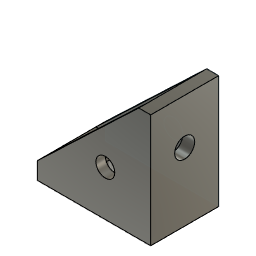
2020_CornerCube-18mm (Autodesk Fusion 360 design; units mm, degrees)
Autodesk Fusion 360 part; units mm, degrees
sketch "スケッチ1" plane through (0, 0, 0) normal (1, 0, 0) x (0, 1, 0)
  line L0 (0, 0) -> (0, 30)
  line L1 (0, 0) -> (30, 0)
  line L2 (30, 0) -> (0, 30)
  constraint coincident L0.start L1.start
  constraint vertical L0
  constraint perpendicular L0 L1
sketch "スケッチ2" plane through (0, 0, 0) normal (1, 0, 0) x (0, 1, 0)
  circle A0 centre (20, 12) radius 2.5
  dimension "d3" = 5
  measures "d3" diameter of A0
sketch "スケッチ3" plane through (0, 0, 0) normal (0, 1, 0) x (1, 0, 0)
  line L0 (2.5, -4.5) -> (15, -4.5)
  line L1 (15, -4.5) -> (15, -30)
  line L2 (15, -30) -> (2.5, -30)
  line L3 (2.5, -4.5) -> (2.5, -30)
  constraint horizontal L0
  constraint perpendicular L0 L1
  constraint perpendicular L1 L2
  constraint coincident L2 L3.end
  constraint perpendicular L2 L3
sketch "スケッチ4" plane through (0, 0, 0) normal (0, 0, 1) x (1, 0, 0)
  line L0 (0, 0) -> (30, 0)
  line L1 (30, 0) -> (30, 30)
  line L2 (30, 30) -> (26.836, 30)
  line L3 (0, 0) -> (0, 4.5)
  line L4 (0, 4.5) -> (26.836, 30)
  dimension "d8" = 3.164
  dimension "d9" = 4.5
  constraint coincident L0.start L3.start
  constraint horizontal L0
  constraint perpendicular L0 L1
  constraint perpendicular L1 L2
  constraint perpendicular L0 L3
  measures "d8" distance of L1.end L2.end
  measures "d9" distance of L0.start L3.end
extrude "押し出し4" add sketch "スケッチ4" against normal blind 18
move_body "移動2" bodies 1 to x (1, 0, 0) y (0, 0, 1) z (0, -1, 0) at (0, -18, 0)
sketch "スケッチ5" plane through (0, 0, 0) normal (0, 1, 0) x (-1, 0, 0)
  line L0 (-30, 0) -> (0, 0)
  line L1 (0, 0) -> (0, 4.5)
  line L2 (0, 4.5) -> (-26.836, 30)
  line L3 (-26.836, 30) -> (-30, 30)
  line L4 (-30, 30) -> (-30, 0)
  circle A0 centre (-18, 12) radius 2.5
  dimension "d12" = 5
  measures "d12" diameter of A0
extrude "押し出し5" cut sketch "スケッチ5" against normal blind 18 contours A0
sketch "スケッチ6" plane through (0, 0, 0) normal (0, 1, 0) x (-1, 0, 0)
  circle A0 centre (-18, 12) radius 2.5
  line L0 (-30, 0) -> (0, 0)
  line L1 (0, 0) -> (0, 4.5)
  line L2 (0, 4.5) -> (-26.836, 30)
  line L3 (-26.836, 30) -> (-30, 30)
  line L4 (-30, 30) -> (-30, 0)
sketch "スケッチ7" plane through (-2.2471, 0, 2.3648) normal (-0.688832, 0, 0.724921) x (0, -1, 0)
  line L0 (18, 3.0997) -> (18, 40.1189)
  line L1 (18, 40.1189) -> (0, 40.1189)
  line L2 (0, 40.1189) -> (0, 3.0997)
  line L3 (0, 3.0997) -> (18, 3.0997)
sketch "スケッチ8" plane through (0, 0, 0) normal (1, 0, 0) x (0, 1, 0)
  line L0 (-2.5, 4.5) -> (-15.5, 4.5)
  line L1 (-15.5, 4.5) -> (-15.5, 30)
  line L2 (-15.5, 30) -> (-2.5, 30)
  line L3 (-2.5, 30) -> (-2.5, 4.5)
  constraint horizontal L0
  constraint perpendicular L0 L1
  constraint perpendicular L1 L2
  constraint perpendicular L2 L3
extrude "押し出し6" cut sketch "スケッチ8" along normal blind 26.836
sketch "スケッチ9" plane through (0, 0, 0) normal (0, 1, 0) x (-1, 0, 0)
sketch "スケッチ10" plane through (0, 0, 0) normal (1, 0, 0) x (0, 1, 0)
  circle A0 centre (-9, 18) radius 2.65
  dimension "d17" = 5.3
  measures "d17" diameter of A0
extrude "押し出し7" cut sketch "スケッチ10" along normal blind 30
sketch "スケッチ11" plane through (0, 0, 0) normal (0, 1, 0) x (-1, 0, 0)
sketch "スケッチ12" plane through (0, 0, 0) normal (0, 0, 1) x (1, 0, 0)
  circle A0 centre (20, -9) radius 2.65
  circle A1 centre (12, -9) radius 2.65
  dimension "d20" = 5.3
  dimension "d21" = 5.3
  measures "d20" diameter of A0
  measures "d21" diameter of A1
extrude "押し出し8" cut sketch "スケッチ12" along normal blind 4.5
